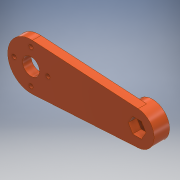
# Autodesk Inventor part: 04-01-Качалка
Saved by Autodesk Inventor 2018 (Build 220112000, 112)
## iProperties
Part Number: 04-01-Качалка
Material: Типовые
Document SubType Name: Modeling
Designer: sbnnl
Density: 1 g/cm^3
Appearance: Гладкий — светло-оранжевый
Author: sbnnl
Autodesk Inventor part; units mm, degrees
ref_plane "YZ Plane" through (0, 0, 0) normal (1, 0, 0) x (0, 1, 0)
ref_plane "XZ Plane" through (0, 0, 0) normal (0, 1, 0) x (-1, 0, 0)
ref_plane "XY Plane" through (0, 0, 0) normal (0, 0, 1) x (1, 0, 0)
sketch "Эскиз1" plane through (0, 0, 0) normal (0, 1, 0) x (-1, 0, 0)
  arc A0 (-0.66, -10.9802) -> (-0.66, 10.9802) centre (0, 0) ccw
  line L0 (0, 0) -> (-50, 0) construction
  arc A1 (-50.48, 7.9856) -> (-50.48, -7.9856) centre (-50, 0) ccw
  circle A2 centre (-50, 0) radius 2.25
  circle A3 centre (0, 0) radius 4
  line L1 (-0.66, 10.9802) -> (-50.48, 7.9856)
  line L2 (-50.48, -7.9856) -> (-0.66, -10.9802)
  line L3 (0, 14.7919) -> (0, -15.3295) construction
  circle A4 centre (0, 8) radius 1
  circle A5 centre (-8, 0) radius 1
  circle A6 centre (0, -8) radius 1
  circle A7 centre (8, 0) radius 1
  dimension "d0" = 22
  dimension "d1" = 16
  dimension "d2" = 4.5
  dimension "d3" = 8
  dimension "d4" = 50
  dimension "d7" = 2
  dimension "d8" = 8
  dimension "d25" = 360
  constraints: 8 centre point, 8 end point, 4 coincident, 4 point on circle, 4 tangent, 2 point on line, 1 horizontal, 1 vertical, 9 other
  measures "d0" diameter of A0
  measures "d1" diameter of A1
  measures "d2" diameter of A2
  measures "d3" diameter of A3
  measures "d4" distance of L0.end point (0, 0)
  measures "d7" diameter of A4
  measures "d8" distance of A4.centre point (0, 0)
extrude "Выдавливание1" add sketch "Эскиз1" along normal blind 4
sketch "Эскиз3" plane through (0, 0, 0) normal (0, -1, 0) x (1, 0, 0)
  circle A0 centre (50, 0) radius 2.25 projected
  circle A1 centre (50, 0) radius 8
  arc A2 (50.48, -7.9856) -> (50.48, 7.9856) centre (50, 0) ccw projected
  point P0 (0, 0)
  constraints: 1 centre point, 1 coincident, 1 concentric
extrude "Выдавливание3" add sketch "Эскиз3" against normal blind 7.25
sketch "Эскиз5" plane through (0, 4, 0) normal (0, 1, 0) x (1, 0, 0)
  circle A0 centre (50, 0) radius 2.25 projected
  line L0 (54.1569, 0) -> (52.0785, -3.6)
  line L1 (52.0785, -3.6) -> (47.9215, -3.6)
  line L2 (47.9215, -3.6) -> (45.8431, 0)
  line L3 (45.8431, 0) -> (47.9215, 3.6)
  line L4 (47.9215, 3.6) -> (52.0785, 3.6)
  line L5 (52.0785, 3.6) -> (54.1569, 0)
  point P0 (0, 0)
  dimension "d20" = 7.2
  dimension "d31" = 4.1569
  dimension "d32" = 3.6
  dimension "d33" = 50
  constraints: 12 end point, 1 coincident, 1 horizontal, 13 other
  measures "d20" distance between parallel lines of L4 L1
  measures "d31" distance of L0.end L1.end
  measures "d32" distance from line of L0 A0.centre
  measures "d33" distance of A0.centre point (0, 0)
extrude "Выдавливание8" cut sketch "Эскиз5" against normal blind 4
sketch "Эскиз8" plane through (50, 7.25, 0) normal (0, 1, 0) x (1, 0, 0)
  circle A0 centre (0, 0) radius 2.25 projected
  circle A1 centre (0, 0) radius 2.2361
  circle A2 centre (0, 0) radius 3.5
  point P0 (-50, 0)
  dimension "d38" = 7
  constraints: 2 centre point, 2 coincident
  measures "d38" diameter of A2
extrude "Выдавливание9" add sketch "Эскиз8" along normal blind 1.3 contours A2
chamfer "Фаска2" distance 1 angle 45 1 edges at (46.5, 8.55, 0)
